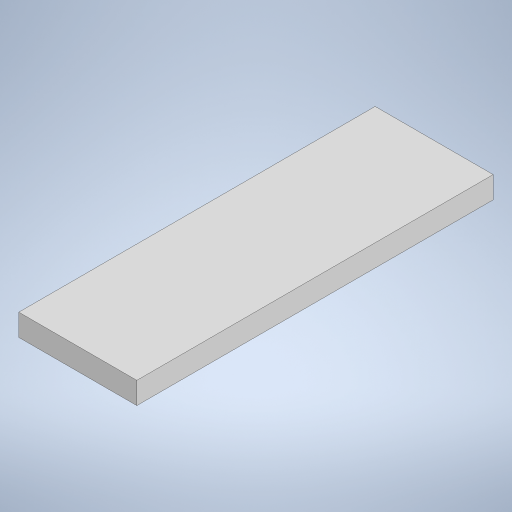
# Autodesk Inventor part: protoboard
Saved by Autodesk Inventor 2023 (Build 270158000, 158)
## iProperties
Created: 2022-11-26
Part Number: protoboard
Material: Genérico
Document SubType Name: Modeling
Designer: inigo
Density: 1 g/cm^3
Appearance: Valor por defecto
Author: inigo
Autodesk Inventor part; units mm, degrees
ref_plane "YZ Plane" through (0, 0, 0) normal (1, 0, 0) x (0, 1, 0)
ref_plane "XZ Plane" through (0, 0, 0) normal (0, 1, 0) x (-1, 0, 0)
ref_plane "XY Plane" through (0, 0, 0) normal (0, 0, 1) x (1, 0, 0)
sketch "Boceto1" plane through (0, 0, 0) normal (0, 1, 0) x (-1, 0, 0)
  line L0 (27, 81.5) -> (-27, 81.5)
  line L1 (-27, 81.5) -> (-27, -81.5)
  line L2 (-27, -81.5) -> (27, -81.5)
  line L3 (27, -81.5) -> (27, 81.5)
  line L4 (27, 81.5) -> (-27, -81.5) construction
  line L5 (-27, 81.5) -> (27, -81.5) construction
  point P0 (0, 0)
  dimension "d0" = 54
  dimension "d1" = 163
  constraints: 12 end point, 2 midpoint, 2 parallel, 1 horizontal, 1 perpendicular
  measures "d0" distance of L2.end L1.end
  measures "d1" distance of L1.end L0.end
extrude "Extrusión1" add sketch "Boceto1" along normal blind 10
